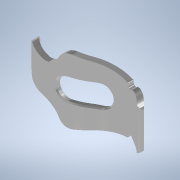
# Autodesk Inventor part: YTP-AP-E15-R1.0
Saved by Autodesk Inventor 2020.4 (Build 244396000, 396)
## iProperties
RuleStatus: InUse
AfterDocNew0: iPropertyEnforcement
BeforeDocSave0: Materialprüfung
Created: 2021-08-29
Part Number: YTP-AP-E15-R1.0
Material: Allgemein
Document SubType Name: Modeling
Designer: Uwe Wieser
Mass: 0.0237232 g
Surface Area: 1.16854 cm^2
Volume: 0.0237232 cm^3
Density: 1 g/cm^3
Appearance: Chrom - poliert
Project: Airbrush
Description: Mitnehmer
Werkstoff: 1.4301
Author: Uwe Wieser
Autodesk Inventor part; units mm, degrees
ref_plane "YZ Plane" through (0, 0, 0) normal (1, 0, 0) x (0, 1, 0)
ref_plane "XZ Plane" through (0, 0, 0) normal (0, 1, 0) x (-1, 0, 0)
ref_plane "XY Plane" through (0, 0, 0) normal (0, 0, 1) x (1, 0, 0)
sketch "Skizze1" plane through (0, 0, 0) normal (0, 0, 1) x (1, 0, 0)
  arc A0 (0, -0.8245) -> (6.5344, -1.6933) centre (3.7628, 2.4681) ccw
  arc A1 (0, 0) -> (6.2573, -1.2772) centre (3.7628, 2.4681) ccw
  arc A2 (11.5, -2.3331) -> (6.5344, -1.6933) centre (8.6493, -4.8686) ccw
  arc A3 (12, -2.1496) -> (6.2573, -1.2772) centre (8.6493, -4.8686) ccw
  line L0 (11.5, -2.3331) -> (12, -2.1496)
  line L1 (0, -6.3359) -> (0, 3.9355) projected
  line L2 (-2.7527, 0) -> (14.6557, 0) projected
  line L3 (0, -0.8245) -> (0, 0)
  dimension "d0" = 0.5
  dimension "d1" = 3.8151
  dimension "d2" = 4.3151
  dimension "d3" = 4.5
  dimension "d4" = 5
  dimension "d31" = 12
  dimension "d33" = 4.8686
  dimension "d34" = 2.4681
  dimension "d44" = 0.5
  constraints: 8 point on circle, 4 centre point, 4 end point, 3 point on line, 1 coincident, 1 collinear, 1 concentric, 1 tangent
  measures "d0" horizontal distance of L0.start L0.end
  measures "d1" radius of A2
  measures "d2" radius of A3
  measures "d3" radius of A1
  measures "d4" radius of A0
  measures "d31" distance from line of L1 L0.end
  measures "d33" distance from line of L2 A2.centre
  measures "d34" distance from line of L2 A0.centre
  measures "d44" radial gap between concentric circles of A1 A0
extrude "Extrusion1" add sketch "Skizze1" along normal mid plane 10
sketch "Skizze2" plane through (0, 0, 0) normal (0, 1, 0) x (-1, 0, 0)
  line L0 (-7, 1) -> (-5, 1)
  spline S0 degree 3 poles (-4.4532, 2.6802) (-4.4614, 2.6893) (-4.4698, 2.6982) (-4.5673, 2.7982) (-4.6799, 2.877) (-4.9286, 2.9823) (-5.0648, 3.0088) (-5.2569, 3.0088) (-5.3221, 3.0028) (-5.3873, 2.99) knots 0 0 0 0 0.036721 0.036721 0.42457 0.42457 0.81242 0.81242 1 1 1 1
  line L1 (-5.3873, 2.99) -> (-9.3761, 2.2055)
  spline S1 degree 3 poles (-9.3761, 2.2055) (-9.3847, 2.2094) (-9.3939, 2.2124) (-9.4218, 2.2182) (-9.4415, 2.2181) (-9.4738, 2.2105) (-9.4884, 2.2047) (-9.5155, 2.187) (-9.528, 2.1752) (-9.5375, 2.1618) knots 0 0 0 0 0.177135 0.177135 0.518162 0.518162 0.759081 0.759081 1 1 1 1
  line L2 (-9.5375, 2.1618) -> (-9.5375, 1.8263)
  line L3 (-9.5375, 1.8263) -> (-9.8375, 1.8263)
  spline S2 degree 3 poles (-9.8375, 1.8263) (-10.0069, 1.9482) (-10.213, 2.0426) (-10.6615, 2.1328) (-10.9034, 2.1298) (-11.2848, 2.0273) (-11.4419, 1.9631) (-11.6673, 1.8149) (-11.7409, 1.7573) (-11.8787, 1.6263) (-11.9429, 1.553) (-12, 1.4737) knots 0 0 0 0 0.316271 0.316271 0.632542 0.632542 0.816271 0.816271 0.908135 0.908135 1 1 1 1
  line L4 (-12, -1.6263) -> (-12, 1.4737)
  spline S3 degree 3 poles (-12, -1.6263) (-11.9381, -1.7008) (-11.8695, -1.7688) (-11.7243, -1.8889) (-11.6476, -1.9407) (-11.4145, -2.0718) (-11.2547, -2.1245) (-10.8706, -2.1996) (-10.6312, -2.186) (-10.194, -2.0659) (-9.9966, -1.9585) (-9.8375, -1.8263) knots 0 0 0 0 0.091865 0.091865 0.183729 0.183729 0.367458 0.367458 0.683729 0.683729 1 1 1 1
  line L5 (-9.5375, -1.8263) -> (-9.8375, -1.8263)
  line L6 (-9.5375, -2.1618) -> (-9.5375, -1.8263)
  spline S4 degree 3 poles (-9.5375, -2.1618) (-9.5375, -2.1868) (-9.5325, -2.2124) (-9.5145, -2.2581) (-9.5015, -2.2782) (-9.4682, -2.316) (-9.4439, -2.3335) (-9.4042, -2.3509) (-9.3901, -2.3552) (-9.3761, -2.358) knots 0 0 0 0 0.240919 0.240919 0.481838 0.481838 0.822865 0.822865 1 1 1 1
  line L7 (-5.3873, -3.1426) -> (-9.3761, -2.358)
  spline S5 degree 3 poles (-5.3873, -3.1426) (-5.3221, -3.1554) (-5.2569, -3.1613) (-5.0648, -3.1613) (-4.9286, -3.1348) (-4.6799, -3.0295) (-4.5673, -2.9507) (-4.4698, -2.8507) (-4.4614, -2.8419) (-4.4532, -2.8328) knots 0 0 0 0 0.18758 0.18758 0.57543 0.57543 0.963279 0.963279 1 1 1 1
  line L8 (-5, -1) -> (-7, -1)
  spline S6 degree 3 poles (-4.4532, -2.8328) (-4.3895, -2.7625) (-4.3319, -2.6779) (-4.2884, -2.585) knots 0 0 0 0 1 1 1 1
  spline S7 degree 3 poles (-2.7032, -1.5763) (-2.9261, -1.5763) (-3.1619, -1.6214) (-3.5925, -1.8011) (-3.7875, -1.9355) (-4.0786, -2.2269) (-4.2005, -2.3969) (-4.2884, -2.585) knots 0 0 0 0 0.345719 0.345719 0.691437 0.691437 1 1 1 1
  line L9 (-1.3066, -1.5763) -> (-2.7032, -1.5763)
  spline S8 degree 3 poles (-1.3066, -1.5763) (-1.1258, -1.5789) (-0.934, -1.5561) (-0.5874, -1.4341) (-0.4325, -1.3343) (-0.2195, -1.1045) (-0.1383, -0.9745) (-0.0299, -0.6854) (-0.0022, -0.5264) (0, -0.3763) knots 0 0 0 0 0.279446 0.279446 0.558892 0.558892 0.779446 0.779446 1 1 1 1
  line L10 (0, -0.3763) -> (0, 0.3763)
  spline S9 degree 3 poles (0, 0.3763) (-0.0116, 0.5175) (-0.0477, 0.6655) (-0.1682, 0.9309) (-0.2529, 1.0483) (-0.468, 1.2512) (-0.6202, 1.3354) (-0.9544, 1.4283) (-1.1365, 1.4377) (-1.3066, 1.4237) knots 0 0 0 0 0.220554 0.220554 0.441108 0.441108 0.720554 0.720554 1 1 1 1
  line L11 (-1.3066, 1.4237) -> (-2.7032, 1.4237)
  spline S10 degree 3 poles (-2.7032, 1.4237) (-2.9261, 1.4237) (-3.1619, 1.4689) (-3.5925, 1.6486) (-3.7875, 1.783) (-4.0786, 2.0744) (-4.2005, 2.2443) (-4.2884, 2.4324) knots 0 0 0 0 0.345719 0.345719 0.691437 0.691437 1 1 1 1
  spline S11 degree 3 poles (-4.2884, 2.4324) (-4.3319, 2.5254) (-4.3895, 2.61) (-4.4532, 2.6802) knots 0 0 0 0 1 1 1 1
  line L12 (2.7739, 0) -> (-14.568, 0)
  line L13 (-12, -5) -> (-12, 5)
  arc A0 (-5, -1) -> (-5, 1) centre (-5, 0) ccw
  line L14 (0, -7) -> (0, 7)
  line L15 (-12, 5) -> (0, 5)
  line L16 (-12, -5) -> (0, -5)
  arc A1 (-7, 1) -> (-7, -1) centre (-7, 0) ccw
  point P0 (0, 0)
  point P1 (-10.0375, 3.1737)
  point P2 (-12, -0.0763)
  point P3 (0, 0)
  point P4 (-12, 1.4737)
  point P5 (-4.4532, -2.8328)
  dimension "d36" = 1
  dimension "d37" = 5
  dimension "d38" = 78.873
  dimension "d40" = 78.873
  dimension "d41" = 2
  dimension "d42" = 1
  dimension "d43" = 2
  constraints: 28 end point, 5 point on line, 4 point on circle, 2 centre point, 2 midpoint, 2 perpendicular, 1 symmetric about line, 30 other
  measures "d36" radius of A0
  measures "d37" distance from line of L14 A0.centre
  measures "d38" angle of L13 L7
  measures "d40" angle of L13 L1
  measures "d41" distance of A0.centre A1.centre
  measures "d42" radius of A1
  measures "d43" distance between parallel lines of L8 L0
extrude "Extrusion2" cut sketch "Skizze2" against normal through all contours L0 A0 L12 A1 | L12 A0 L8 A1 | S3 L5 L6 S4 L7 S5 S6 S7 L9 S8 L14 L16 L13 | L13 L15 L14 S9 L11 S10 S11 S0 L1 S1 L2 L3 S2
fillet "Rundung1" radius 0.2 1 edges at (12, -2.1496, -0.0763)
fillet "Rundung2" radius 0.2 1 edges at (11.5, -2.3331, -0.0505)
fillet "Rundung3" radius 0.2 2 edges at (9.5375, -0.9021, -1.8263) (9.5375, -0.9021, 1.8263)
chamfer "Fase2" distance 0.1 angle 45 10 edges at (6.7626, -1.5527, -1) (6.7626, -1.5527, 1) (6.619, -1.061, 1) (6.619, -1.061, -1) (4, -2.0256, 0) (5.6511, -1.6165, -1) (5.6511, -1.6165, 1) (5.7961, -2.0997, 1) (4, -2.5262, 0) (5.7961, -2.0997, -1)
